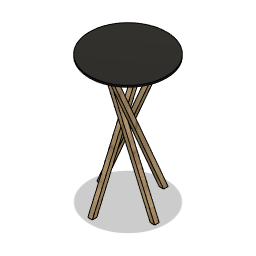
bar v6 (Autodesk Fusion 360 design; units mm, degrees)
Autodesk Fusion 360 part; units mm, degrees
sketch "スケッチ1" plane through (0, 0, 0) normal (0, 1, 0) x (1, 0, 0)
  line L0 (-17.5, -17.5) -> (17.5, -17.5)
  line L1 (17.5, -17.5) -> (17.5, 17.5)
  line L2 (17.5, 17.5) -> (-17.5, 17.5)
  line L3 (-17.5, 17.5) -> (-17.5, -17.5)
  line L4 (-17.5, -17.5) -> (17.5, 17.5) construction
  line L5 (17.5, -17.5) -> (-17.5, 17.5) construction
  dimension "d1" = 35
  dimension "d2" = 35
  constraint perpendicular L0 L1
  constraint parallel L0 L2
  constraint parallel L1 L3
  constraint horizontal L0
  constraint coincident L4 origin
  constraint coincident L5 origin
  measures "d1" distance of L1.end L2.end
  measures "d2" distance of L0.end L1.end
extrude "押し出し1" add sketch "スケッチ1" along normal blind 988 makes body 1
sketch "スケッチ2" plane through (0, 988, 0) normal (0, 1, 0) x (-1, 0, 0)
  line L0 (17.5, -17.5) -> (17.5, 17.5)
  line L1 (17.5, 17.5) -> (-17.5, 17.5)
  line L2 (-17.5, 17.5) -> (-17.5, -17.5)
  line L3 (-17.5, -17.5) -> (17.5, -17.5)
  circle A0 centre (0, 0) radius 300
  dimension "d5" = 600
  constraint coincident A0.centre origin
  measures "d5" diameter of A0
extrude "押し出し2" add sketch "スケッチ2" along normal blind 12 separate body makes body 2
extrude "押し出し3" add 1 faces at (5.8333, 992, -17.5) along direction (0, 0, 1) blind 35 on bodies 2 bodies 2
sketch "スケッチ3" plane through (0, 988, 0) normal (0, 1, 0) x (-1, 0, 0)
  line L0 (17.5, -17.5) -> (17.5, 17.5)
  line L1 (17.5, 17.5) -> (-17.5, 17.5)
  line L2 (-17.5, 17.5) -> (-17.5, -17.5)
  line L3 (-17.5, -17.5) -> (17.5, -17.5)
  line L4 (45, 45) -> (-45, 45)
  line L5 (-45, 45) -> (-45, -45)
  line L6 (-45, -45) -> (45, -45)
  line L7 (45, -45) -> (45, 45)
  line L8 (45, 45) -> (-45, -45) construction
  line L9 (-45, 45) -> (45, -45) construction
  line L10 (45, 45) -> (10, 45)
  line L11 (10, 45) -> (10, 10)
  line L12 (10, 10) -> (45, 10)
  line L13 (45, 10) -> (45, 45)
  line L14 (45, -45) -> (10, -45)
  line L15 (10, -45) -> (10, -10)
  line L16 (10, -10) -> (45, -10)
  line L17 (45, -10) -> (45, -45)
  line L18 (-45, 45) -> (-10, 45)
  line L19 (-10, 45) -> (-10, 10)
  line L20 (-10, 10) -> (-45, 10)
  line L21 (-45, 10) -> (-45, 45)
  line L22 (-45, -45) -> (-10, -45)
  line L23 (-10, -45) -> (-10, -10)
  line L24 (-10, -10) -> (-45, -10)
  line L25 (-45, -10) -> (-45, -45)
  dimension "d10" = 90
  dimension "d11" = 90
  dimension "d12" = 35
  dimension "d13" = 35
  dimension "d14" = 35
  dimension "d15" = 35
  dimension "d16" = 35
  dimension "d17" = 35
  dimension "d18" = 35
  dimension "d19" = 35
  constraint perpendicular L4 L5
  constraint parallel L4 L6
  constraint parallel L5 L7
  constraint horizontal L4
  constraint coincident L8 origin
  constraint coincident L9 origin
  constraint horizontal L10
  constraint vertical L11
  constraint horizontal L12
  constraint vertical L13
  constraint horizontal L14
  constraint vertical L15
  constraint horizontal L16
  constraint vertical L17
  constraint horizontal L18
  constraint vertical L19
  constraint horizontal L20
  constraint vertical L21
  constraint horizontal L22
  constraint vertical L23
  constraint horizontal L24
  constraint vertical L25
  measures "d10" distance of L5.end L6.end
  measures "d11" distance of L4.end L5.end
  measures "d12" distance of L4.start L10.end
  measures "d13" distance of L4.start L12.end
  measures "d14" distance of L6.end L14.end
  measures "d15" distance of L6.end L16.end
  measures "d16" distance of L4.end L18.end
  measures "d17" distance of L4.end L20.end
  measures "d18" distance of L5.end L24.end
  measures "d19" distance of L5.end L22.end
extrude "押し出し4" add sketch "スケッチ3" against normal blind 988 contours L1 L2 L19 L20 | L1 L2 L4 L5 L18 L19 L20 L21 bodies 2
move_face "面を移動1" to x (0.965926, 0.258819, 0) y (-0.258819, 0.965926, 0) z (0, 0, 1) at (1.5333, -11.6469, 0) 1 faces at (33.3333, 0, 33.3333) on bodies 2
sketch "スケッチ4" plane through (0, 0, 0) normal (0, 1, 0) x (1, 0, 0)
  line L0 (300, 500) -> (335, 500)
  line L1 (335, 500) -> (335, 465)
  line L2 (335, 465) -> (300, 465)
  line L3 (300, 465) -> (300, 500)
  dimension "d22" = 35
  dimension "d23" = 35
  constraint horizontal L0
  constraint vertical L1
  constraint horizontal L2
  constraint vertical L3
  measures "d22" distance of L0.start L0.end
  measures "d23" distance of L0.start L2.end
sketch "スケッチ5" plane through (300, 0, 0) normal (-1, 0, 0) x (0, 0, 1)
  line L0 (-500, 0) -> (-465, 0)
  line L1 (-465, 0) -> (-465, 1022.8)
  line L2 (-465, 1022.8) -> (-500, 1022.8)
  line L3 (-500, 1022.8) -> (-500, 0)
  line L4 (-500, 1022.8) -> (-463.4899, 1013.0171)
  line L5 (-500, 1022.8) -> (-462.2019, 1022.8) construction
  line L6 (-465, 0) -> (-500, 9.3782)
  line L7 (-465, 0) -> (-428.7653, 0) construction
  dimension "d26" = 15
  dimension "d27" = 165
  constraint horizontal L5
  constraint coincident L2.end L3.start
  constraint horizontal L7
  constraint coincident L0.end L1.start
  constraint coincident L3 L6.end
  measures "d26" angle of L4 L5
  measures "d27" angle of L6 L7
sketch "スケッチ6" plane through (300, 0, 0) normal (-1, 0, 0) x (0, 0, 1)
  line L0 (-500, 9.3782) -> (-465, 0)
  line L1 (-465, 0) -> (-465, 1022.8)
  line L2 (-465, 1022.8) -> (-500, 1022.8)
  line L3 (-500, 1022.8) -> (-500, 9.3782)
  line L4 (-500, 1022.8) -> (-459.6784, 1011.9959)
  line L5 (-500, 1022.8) -> (-458.2561, 1022.8) construction
  dimension "d30" = 15
  constraint horizontal L5
  constraint coincident L2.end L3.start
  measures "d30" angle of L4 L5
extrude "押し出し8" cut 1 faces at (10, 655.5406, 33.3333) along direction (1, 0, 0) blind 40 on bodies 2 bodies 2
sketch "スケッチ7" plane through (0, 0, 0) normal (1, 0, 0) x (0, 0, -1)
  line L0 (0, 0) -> (-461, 0)
  line L1 (-461, 0) -> (-461, 988)
  line L2 (-461, 988) -> (0, 988)
  line L3 (0, 988) -> (0, 0)
  line L4 (-461, 988) -> (-426, 988)
  line L5 (0, 0) -> (-35, 0)
  line L6 (-461, 988) -> (-35, 0)
  line L7 (-426, 988) -> (0, 0)
  dimension "d41" = 988
  dimension "d42" = 461
  dimension "d43" = 35
  dimension "d44" = 35
  constraint horizontal L0
  constraint vertical L1
  constraint horizontal L2
  constraint vertical L3
  constraint coincident L0.start L3.end
  constraint perpendicular L1 L4
  constraint horizontal L5
  measures "d41" distance of L0.start L2.end
  measures "d42" distance of L0.start L0.end
  measures "d43" distance of L1.end L4.end
  measures "d44" distance of L0.start L5.end
extrude "押し出し9" add sketch "スケッチ7" along normal blind 35 separate body contours L0 L2 L4 L5 L6 L7 makes body 3
move_body "移動4" bodies 3 to x (1, 0, 0) y (0, 1, 0) z (0, 0, 1) at (0, 0, -261)
copy_body "ボディのコピーと貼り付け1" bodies 3 makes body 4
move_body "移動5" bodies 4 to x (0, 0, -1) y (0, 1, 0) z (1, 0, 0) at (0, 0, 0)
copy_body "ボディのコピーと貼り付け2" bodies 4 makes body 5
move_body "移動6" bodies 5 to x (0, 0, -1) y (0, 1, 0) z (1, 0, 0) at (0, 0, 0)
copy_body "ボディのコピーと貼り付け3" bodies 5 makes body 6
move_body "移動7" bodies 6 to x (0, 0, -1) y (0, 1, 0) z (1, 0, 0) at (0, 0, 0)
move_body "移動8" bodies 6 to x (1, 0, 0) y (0, 1, 0) z (0, 0, 1) at (0, 0, 17.5)
move_face "面を移動2" by (0, 0, -17.5) 1 faces at (23, 658.6667, -23.3333) on bodies 4
move_face "面を移動3" by (17.5, 0, 0) 1 faces at (23.3333, 658.6667, 58) on bodies 3
move_body "移動9" bodies 3 to x (1, 0, 0) y (0, 1, 0) z (0, 0, 1) at (17.5, 0, 0)
move_body "移動10" bodies 5 to x (1, 0, 0) y (0, 1, 0) z (0, 0, 1) at (-17.5, 0, 0)
move_body "移動11" bodies 4 to x (1, 0, 0) y (0, 1, 0) z (0, 0, 1) at (0, 0, -17.5)
sketch "スケッチ8" plane through (0, 988, 0) normal (0, -1, 0) x (1, 0, 0)
  circle A0 centre (0, 0) radius 300
  line L0 (-17.5, -17.5) -> (17.5, -17.5)
  line L1 (17.5, -17.5) -> (17.5, 17.5)
  line L2 (17.5, 17.5) -> (-17.5, 17.5)
  line L3 (-17.5, 17.5) -> (-17.5, -17.5)
  line L4 (-17.5, -17.5) -> (17.5, 17.5) construction
  line L5 (17.5, -17.5) -> (-17.5, 17.5) construction
  dimension "d71" = 35
  dimension "d72" = 35
  constraint perpendicular L0 L1
  constraint parallel L0 L2
  constraint parallel L1 L3
  constraint horizontal L0
  constraint coincident L4 A0.centre
  constraint coincident L5 A0.centre
  constraint coincident A0.centre origin
  measures "d71" distance of L0.end L1.end
  measures "d72" distance of L1.end L2.end
sketch "スケッチ11" plane through (0, 0, 0) normal (0, 1, 0) x (1, 0, 0)
  line L0 (17.5, -17.5) -> (-17.5, -17.5)
  line L1 (-17.5, -17.5) -> (-17.5, 17.5)
  line L2 (-17.5, 17.5) -> (17.5, 17.5)
  line L3 (17.5, 17.5) -> (17.5, -17.5)
  line L4 (17.5, -17.5) -> (-17.5, 17.5) construction
  line L5 (-17.5, -17.5) -> (17.5, 17.5) construction
  dimension "d89" = 35
  dimension "d90" = 35
  constraint horizontal L0
  constraint perpendicular L0 L1
  constraint parallel L0 L2
  constraint parallel L1 L3
  constraint coincident L4 origin
  constraint coincident L5 origin
  measures "d89" distance of L1.end L2.end
  measures "d90" distance of L0.end L1.end
extrude "押し出し15" add sketch "スケッチ11" along normal blind 70 separate body makes body 7
move_body "移動17" bodies 7 to x (1, 0, 0) y (0, 1, 0) z (0, 0, 1) at (0, 530, 0)
extrude "押し出し10" [suppressed]
other "面を置換1"
split "分割1" [suppressed]
extrude "押し出し11" [suppressed]
sketch "スケッチ9" plane through (0, 0, 17.5) normal (0, 0, -1) x (-1, 0, 0)
  line L0 (17.5, 564.7371) -> (200, 988)
  line L1 (200, 988) -> (165, 988)
  line L2 (165, 988) -> (-17.5, 564.7371)
  line L3 (-17.5, 564.7371) -> (-261, 0)
  line L4 (-261, 0) -> (-226, 0)
  line L5 (-226, 0) -> (17.5, 564.7371)
  line L6 (-17.5, 564.7371) -> (17.5, 564.7371)
  line L7 (17.5, 564.7371) -> (17.5, 599.7371)
  line L8 (17.5, 599.7371) -> (-17.5, 599.7371)
  line L9 (-17.5, 599.7371) -> (-17.5, 564.7371)
  dimension "d77" = 35
  dimension "d78" = 35
  constraint horizontal L6
  constraint vertical L7
  constraint horizontal L8
  constraint vertical L9
  constraint coincident L2.end L3.start
  measures "d77" distance of L2.end L0.start
  measures "d78" distance of L2.end L8.end
extrude "押し出し12" [suppressed]
move_body "移動12" [suppressed]
sketch "スケッチ10" plane through (0, 0, 0) normal (0, 1, 0) x (1, 0, 0)
  line L0 (0, 0) -> (250, 0)
  line L1 (250, 0) -> (250, -35)
  line L2 (250, -35) -> (0, -35)
  line L3 (0, -35) -> (0, 0)
  dimension "d81" = 35
  dimension "d82" = 250
  constraint horizontal L0
  constraint vertical L1
  constraint horizontal L2
  constraint vertical L3
  constraint coincident L0.start L3.end
  measures "d81" distance of L0.start L2.end
  measures "d82" distance of L0.start L0.end
extrude "押し出し13" [suppressed]
move_body "移動13" [suppressed]
copy_body "ボディのコピーと貼り付け4" [suppressed]
move_body "移動14" [suppressed]
copy_body "ボディのコピーと貼り付け5" [suppressed]
move_body "移動15" [suppressed]
combine "結合1" [suppressed]
extrude "押し出し14" [suppressed]
moveface "面を移動4" [suppressed]
move_body "移動16" [suppressed]
hidden bodies 1
named bodies: "足案1", "天板", "脚1", "脚2", "脚3", "脚4", "足案2"
